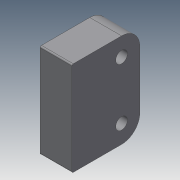
# Autodesk Inventor part: Standard
Saved by Autodesk Inventor 2020.3 (Build 243373000, 373)
## iProperties
RuleStatus: InUse
AfterDocSave0: file://Part Number Cleaner
Created: 2023-01-18
Material: Generic
Catalog Web Link: https://www.janelia.org/
Vendor: HHMI: JRC - jET
Document SubType Name: Modeling
Designer: arnoldj
Density: 1 g/cm^3
Appearance: Default
DESIGN DEPARTMENT: HHMI: JRC - jET
ALTERED ITEM PART NUMBER: N/A
ALTERED ITEM VENDOR: N/A
ALTERED ITEM DESCRIPTION: N/A
Title: Standard
Author: arnoldj
Revision Number: 0
Autodesk Inventor part; units mm, degrees
ref_plane "YZ Plane" through (0, 0, 0) normal (1, 0, 0) x (0, 1, 0)
ref_plane "XZ Plane" through (0, 0, 0) normal (0, 1, 0) x (-1, 0, 0)
ref_plane "XY Plane" through (0, 0, 0) normal (0, 0, 1) x (1, 0, 0)
sketch "Sketch1" plane through (0, 0, 0) normal (1, 0, 0) x (0, 1, 0)
  line L0 (10.75, 26) -> (-6.5, 26)
  arc A0 (-6.5, 26) -> (-7, 25.5) centre (-6.5, 25.5) ccw
  line L1 (-7, 25.5) -> (-7, 7)
  arc A1 (-7, 7) -> (0, 0) centre (0, 7) ccw
  line L2 (0, 0) -> (22, 0)
  arc A2 (22, 0) -> (29, 7) centre (22, 7) ccw
  line L3 (29, 7) -> (29, 25.5)
  arc A3 (29, 25.5) -> (28.5, 26) centre (28.5, 25.5) ccw
  line L4 (28.5, 26) -> (-6.5, 26)
  circle A4 centre (0, 7) radius 2.25
  circle A5 centre (22, 7) radius 2.25
  point P0 (0, 0)
  point P1 (-7, 7)
  point P2 (0, 0)
  constraints: 10 end point, 8 point on circle, 6 centre point
extrude "Extrusion1" add sketch "Sketch1" along normal blind 12.192
body "Solid1"
